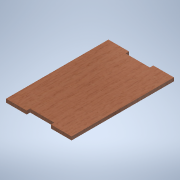
# Autodesk Inventor part: schuine plaat
Saved by Autodesk Inventor 2021 (Build 250183000, 183)
## iProperties
Manager: Pierloot J.
Company: Emmaüs Bovenbouw Aalter
Created: 2021-01-26
Part Number: schuine plaat
Material: S235
Catalog Web Link: http://emmausbovenbouw.op-weg.be/
Vendor: Emmaüsinstituut Bovenbouw Aalter
Document SubType Name: Modeling
Designer: iskhak.tchuytiyev
Engineer: Pierloot J.
Manufacturer: Standard
Standards Organization: Custom
Density: 7.86 g/cm^3
Appearance: White Oak - Natural Medium Gloss
Title: Algemene titel
Subject: Specifieke titel
Author: iskhak.tchuytiyev
Keywords: Ruwe Ø xxxxx
Comments: Opmerking
Autodesk Inventor part; units mm, degrees
ref_plane "YZ Plane" through (0, 0, 0) normal (1, 0, 0) x (0, 1, 0)
ref_plane "XZ Plane" through (0, 0, 0) normal (0, 1, 0) x (-1, 0, 0)
ref_plane "XY Plane" through (0, 0, 0) normal (0, 0, 1) x (1, 0, 0)
sketch "Sketch1" plane through (0, 0, 0) normal (0, 0, 1) x (1, 0, 0)
  line L0 (0, 2.8582) -> (0, -2.8582) construction
  line L1 (-5.7775, 0) -> (5.7775, 0) construction
  line L2 (0, 0) -> (96, 0)
  line L3 (96, 0) -> (96, -150)
  line L4 (96, -150) -> (0, -150)
  line L5 (0, -150) -> (0, 0)
  line L6 (0, 0) -> (30.25, 0)
  line L7 (30.25, 0) -> (66, 0)
  line L8 (0, -150) -> (30.25, -150)
  line L9 (30.25, 0) -> (65.75, 0)
  line L10 (65.75, 0) -> (65.75, -5)
  line L11 (65.75, -5) -> (30.25, -5)
  line L12 (30.25, -5) -> (30.25, 0)
  line L13 (30.25, -150) -> (65.75, -150)
  line L14 (65.75, -150) -> (65.75, -145)
  line L15 (65.75, -145) -> (30.25, -145)
  line L16 (30.25, -145) -> (30.25, -150)
  point P0 (65.75, 0)
  dimension "d1" = 96
  dimension "d2" = 150
  dimension "d3" = 30.25
  dimension "d5" = 30.25
  dimension "d7" = 35.5
  dimension "d8" = 5
  dimension "d9" = 35.5
  dimension "d10" = 5
  dimension "d13" = 30.25
  constraints: 34 end point, 6 parallel, 4 horizontal, 3 perpendicular, 3 point on line, 2 midpoint, 1 vertical
  measures "d1" distance of L3.end L4.end
  measures "d2" distance of L2.end L3.end
  measures "d3" distance of L2.start L6.end
  measures "d5" distance of L4.end L8.end
  measures "d7" distance of L10.end L11.end
  measures "d8" distance of L9.end L10.end
  measures "d9" distance of L15.end L14.end
  measures "d10" distance of L14.end L13.end
  measures "d13" distance between parallel lines of L3 L10
extrude "Extrusion1" add sketch "Sketch1" along normal blind 5 contours L2 L12 L11 L10 L3 L4 L14 L15 L16 L5
body "Solid1"
